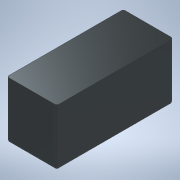
# Autodesk Inventor part: solar_power_buffer_battery
Saved by Autodesk Inventor 2020 (Build 240168000, 168)
## iProperties
Created: 2022-08-31
Part Number: solar_power_buffer_battery
Material: Iron, Ductile
Document SubType Name: Modeling
Designer: Intuito_PC
Density: 7.15 g/cm^3
Appearance: Iron Gray
Author: Intuito_PC
Autodesk Inventor part; units mm, degrees
ref_plane "YZ Plane" through (0, 0, 0) normal (1, 0, 0) x (0, 1, 0)
ref_plane "XZ Plane" through (0, 0, 0) normal (0, 1, 0) x (-1, 0, 0)
ref_plane "XY Plane" through (0, 0, 0) normal (0, 0, 1) x (1, 0, 0)
sketch "Sketch1" plane through (0, 0, 0) normal (0, 0, 1) x (1, 0, 0)
  line L0 (0, 0) -> (-75, 0)
  line L1 (-75, 0) -> (-75, 85)
  line L2 (-75, 85) -> (0, 85)
  line L3 (0, 85) -> (0, 0)
  dimension "d0" = 75
  dimension "d1" = 85
  constraints: 8 end point, 2 parallel, 1 horizontal, 1 perpendicular
  measures "d0" distance of L1.end L2.end
  measures "d1" distance of L0.end L1.end
extrude "Extrusion1" add sketch "Sketch1" along normal blind 175
fillet "Fillet2" radius 3.175 8 edges at (-75, 42.5, 175) (0, 42.5, 175) (-37.5, 0, 175) (-75, 0, 87.5) (0, 0, 87.5) (0, 42.5, 0) (-37.5, 0, 0) (-75, 42.5, 0)
body "Solid1"
